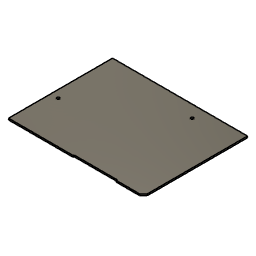
ATX PSU v1 (Autodesk Fusion 360 design; units mm, degrees)
Autodesk Fusion 360 part; units mm, degrees
sketch "Sketch1" plane through (0, 0, 0) normal (0, 1, 0) x (1, 0, 0)
  line L0 (-71.0683, 54.7697) -> (72.9317, 54.7697)
  line L1 (72.9317, 54.7697) -> (72.9317, -52.2303)
  line L2 (-71.0683, -56.2303) -> (-71.0683, 54.7697)
  line L3 (-2.0683, -56.2303) -> (-2.0683, -55.2303)
  line L4 (-2.0683, -55.2303) -> (43.9317, -55.2303)
  line L5 (43.9317, -55.2303) -> (43.9317, -56.2303)
  line L6 (68.9317, -56.2303) -> (43.9317, -56.2303)
  line L7 (-2.0683, -56.2303) -> (-71.0683, -56.2303)
  line L8 (72.9317, -52.2303) -> (68.9317, -52.2303) construction
  line L9 (68.9317, -56.2303) -> (68.9317, -52.2303) construction
  line L10 (68.9317, -56.2303) -> (72.9317, -52.2303)
  circle A0 centre (-63.0683, -11.2303) radius 1.5
  circle A1 centre (26.9317, 41.7697) radius 1.5
  dimension "d3" = 1
  dimension "d4" = 46
  dimension "d5" = 69
  dimension "d6" = 4
  dimension "d8" = 4
  dimension "d11" = 4
  dimension "d14" = 144
  dimension "d17" = 25
  dimension "d18" = 3
  dimension "d19" = 8
  dimension "d20" = 66
  dimension "d21" = 111
  dimension "d23" = 111
  dimension "d24" = 45
  dimension "d25" = 3
  dimension "d26" = 13
  dimension "d27" = 46
  dimension "d28" = 98
  constraint horizontal L0
  constraint parallel L0 L6
  constraint parallel L1 L2
  constraint coincident L3.start L6
  constraint vertical L3
  constraint perpendicular L3 L4
  constraint perpendicular L5 L6
  constraint collinear L6 L7
  constraint perpendicular L1 L8
  measures "d3" distance of L3.start L3.end
  measures "d4" distance of L3.end L4.end
  measures "d5" distance of L2 L3
  measures "d6" distance of L1 L9
  measures "d8" distance of L1 L9
  measures "d11" distance of L6 L8
  measures "d14" distance of L0.start L0.end
  measures "d17" distance of L5.end L6.start
  measures "d18" diameter of A0
  measures "d19" distance of L2 A0.centre
  measures "d20" distance of L0 A0.centre
  measures "d21" distance of L0 L7
  measures "d23" distance of L0 L6
  measures "d24" distance of L7 A0.centre
  measures "d25" diameter of A1
  measures "d26" distance of L0 A1.centre
  measures "d27" distance of L1 A1.centre
  measures "d28" distance of L2 A1.centre
extrude "Extrude1" add sketch "Sketch1" along normal blind 1.6
